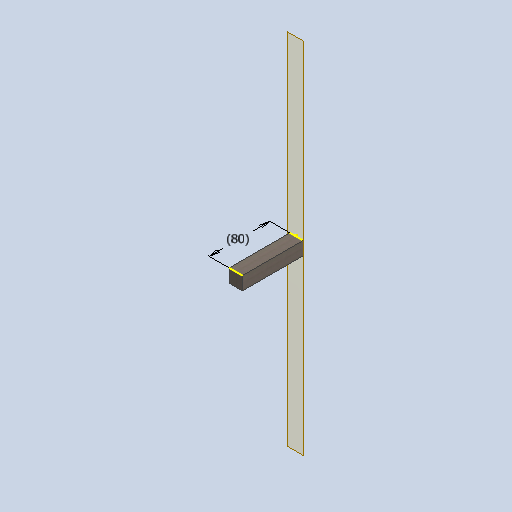
# Autodesk Inventor part: BaseSmall
Saved by Autodesk Inventor 2025.2 (Build 292293000, 293)
## iProperties
Created: 2025-03-06
Part Number: BaseSmall
Material: Wood (Walnut)
Document SubType Name: Modeling
Designer: baolo
Density: 0.55 g/cm^3
Appearance: Walnut
Author: baolo
Autodesk Inventor part; units mm, degrees
ref_plane "YZ Plane" through (0, 0, 0) normal (1, 0, 0) x (0, 1, 0)
ref_plane "XZ Plane" through (0, 0, 0) normal (0, 1, 0) x (-1, 0, 0)
ref_plane "XY Plane" through (0, 0, 0) normal (0, 0, 1) x (1, 0, 0)
ref_plane "Work Plane1" through (0, 0, 0) normal (0, 0, 1) x (1, 0, 0)
sketch "Sketch1" plane through (0, 0, 0) normal (0, 0, 1) x (1, 0, 0)
  line L0 (10, -206.2688) -> (-7.4625, -206.2688)
  line L1 (-7.4625, -206.2688) -> (-7.4625, -223.7313)
  line L2 (-7.4625, -223.7313) -> (10, -223.7313)
  line L3 (10, -223.7313) -> (10, -206.2688)
  line L4 (10, -206.2688) -> (-7.4625, -223.7313) construction
  line L5 (-7.4625, -206.2688) -> (10, -223.7313) construction
  circle A0 centre (292.5375, -215) radius 7.9375 construction
  line L6 (10, -195.95) -> (10, -234.05) construction
  line L7 (10, -234.05) -> (320, -234.05) construction
  line L8 (320, -195.95) -> (320, -234.05) construction
  line L9 (10, -195.95) -> (320, -195.95) construction
  line L10 (-7.4625, -350) -> (10, -350) construction
  point P0 (0, 0)
  point P1 (10, -215)
  constraints: 12 end point, 2 equal length, 2 midpoint, 2 parallel, 1 collinear, 1 perpendicular
extrude "Extrusion1" add sketch "Sketch1" along normal blind 80
sketch "Sketch2" plane through (-7.4625, -206.2688, 0) normal (0, 1, 0) x (1, 0, 0)
  line L0 (17.4625, -80) -> (0, -80) projected
  line L1 (17.4625, 0) -> (0, 0) projected
  point P0 (7.4625, 0)
  dimension "d2" = 80
  measures "d2" distance between parallel lines of L0 L1
body "Solid1"
